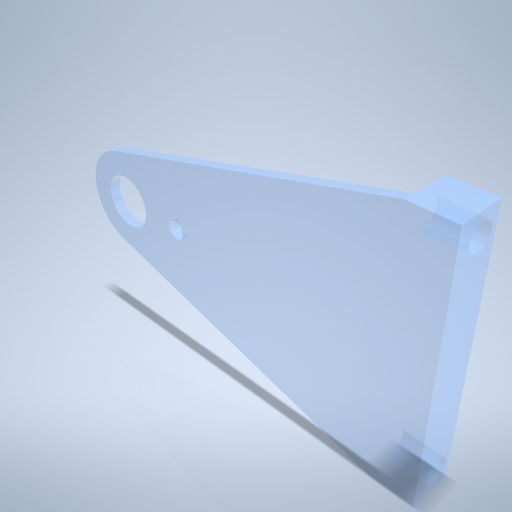
# Autodesk Inventor part: 05
Saved by Autodesk Inventor 2024.2 (Build 282272000, 272)
## iProperties
Created: 2024-05-14
Part Number: 05
Material: Aluminium 6061
Document SubType Name: Modeling
Designer: Fabri
Density: 2.7 g/cm^3
Appearance: Blau - Verglasung
Author: Fabri
Autodesk Inventor part; units mm, degrees
ref_plane "YZ Plane" through (0, 0, 0) normal (1, 0, 0) x (0, 1, 0)
ref_plane "XZ Plane" through (0, 0, 0) normal (0, 1, 0) x (-1, 0, 0)
ref_plane "XY Plane" through (0, 0, 0) normal (0, 0, 1) x (1, 0, 0)
sketch "Skizze1" plane through (0, 0, 0) normal (0, 1, 0) x (-1, 0, 0)
  line L0 (0, 25) -> (0, -25)
  line L1 (0, -25) -> (8, -25)
  line L2 (8, -25) -> (67.4432, -9.1805)
  arc A0 (67.4432, -9.1805) -> (67.4432, 9.1805) centre (65, 0) ccw
  line L3 (67.4432, 9.1805) -> (8, 25)
  line L4 (8, 25) -> (0, 25)
  line L5 (0, 0) -> (65, 0) construction
  dimension "d0" = 9.5
  dimension "d1" = 50
  dimension "d2" = 8
  dimension "d3" = 65
  constraints: 12 end point, 2 point on circle, 1 centre point, 1 horizontal, 1 horizontal alignment, 1 midpoint, 1 parallel, 1 perpendicular, 1 symmetric about line, 1 tangent, 1 vertical, 1 vertical alignment, 1 other
  measures "d0" radius of A0
  measures "d1" distance of L0.start L0.end
  measures "d2" distance of L0.end L1.end
  measures "d3" distance from line of L0 L5.end
extrude "Extrusion1" add sketch "Skizze1" along normal blind 2
sketch "Skizze2" plane through (0, 2, 0) normal (0, 1, 0) x (1, 0, 0)
  line L0 (-67.4432, -9.1805) -> (-8, -25) projected
  line L1 (0, 25) -> (-8, 25) projected
  line L2 (-8, -25) -> (0, -25)
  line L3 (0, -25) -> (0, 25)
  line L4 (0, 25) -> (-8, 25)
  line L5 (-8, 25) -> (-8, -25)
  point P0 (0, 0)
  point P1 (-8, 25)
  constraints: 8 end point, 2 parallel, 1 horizontal, 1 perpendicular
extrude "Extrusion2" add sketch "Skizze2" along normal blind 6.5
sketch "Skizze3" plane through (-8, 2, -25) normal (-1, 0, 0) x (0, 0, 1)
  line L0 (50, -2) -> (0, -2) projected
  line L1 (0, 6.5) -> (50, 6.5) projected
  line L2 (25, 6.5) -> (25, -12.2708) construction
  point P0 (25, -2)
  point P1 (46.124, 3)
  point P2 (3.876, 3)
  dimension "d15" = 5
  dimension "d33" = 42.248
  constraints: 2 end point, 2 midpoint, 1 horizontal alignment, 1 symmetric about line, 1 vertical
  measures "d15" distance from line of L0 point (46.124, 3)
  measures "d33" distance of point (3.876, 3) point (46.124, 3)
hole "Bohrung1" at (-8, 5, 21.124) at (-8, 5, -21.124) direction (1, 0, 0) diameter 5 depth 8
sketch "Skizze4" plane through (0, 2, 0) normal (0, 1, 0) x (1, 0, 0)
  arc A0 (-67.4432, 9.1805) -> (-67.4432, -9.1805) centre (-65, 0) ccw projected
  point P0 (0, 0)
  constraints: 1 coincident
hole "Bohrung2" at (-65, 2, 0) direction (0, -1, 0) diameter 10 depth 2
sketch "Skizze5" plane through (0, 2, 0) normal (0, 1, 0) x (1, 0, 0)
  arc A0 (-67.4432, 9.1805) -> (-67.4432, -9.1805) centre (-65, 0) ccw projected
  point P0 (0, 0)
  point P1 (-51.97, 0)
  point P2 (-74.5, 0)
  dimension "d32" = 13.03
  constraints: 1 horizontal alignment, 1 point on circle
  measures "d32" distance of point (-51.97, 0) A0.centre
hole "Bohrung3" at (-51.97, 2, 0) direction (0, -1, 0) diameter 3.5 depth 2
